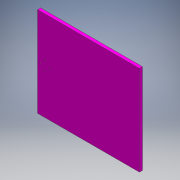
# Autodesk Inventor part: plaque
Saved by Autodesk Inventor 2017 (Build 210142000, 142)
## iProperties
Created: 2017-04-16
Part Number: plaque
Material: Generic
Document SubType Name: Modeling
Designer: franc
Density: 1 g/cm^3
Appearance: Default
Author: franc
Autodesk Inventor part; units mm, degrees
ref_plane "YZ Plane" through (0, 0, 0) normal (1, 0, 0) x (0, 1, 0)
ref_plane "XZ Plane" through (0, 0, 0) normal (0, 1, 0) x (-1, 0, 0)
ref_plane "XY Plane" through (0, 0, 0) normal (0, 0, 1) x (1, 0, 0)
sketch "Sketch1" plane through (0, 0, 0) normal (0, 1, 0) x (-1, 0, 0)
  line L0 (34, 64.6479) -> (-136, 64.6479)
  line L1 (-136, 64.6479) -> (-136, -85.3521)
  line L2 (-136, -85.3521) -> (34, -85.3521)
  line L3 (34, -85.3521) -> (34, 64.6479)
  circle A0 centre (29.5, -10.3521) radius 1
  circle A1 centre (13.5, -10.3521) radius 1
  circle A2 centre (21.5, -18.3521) radius 1
  circle A3 centre (21.5, -2.3521) radius 1
  point P0 (0, 0)
  dimension "d0" = 150
  dimension "d1" = 170
  dimension "d4" = 75
  dimension "d5" = 4.5
  dimension "d6" = 2
  dimension "d16" = 16
  dimension "d17" = 2
  dimension "d18" = 75
  dimension "d19" = 2
  dimension "d20" = 8
  dimension "d21" = 8
  dimension "d22" = 2
  dimension "d23" = 8
  dimension "d24" = 8
  constraints: 8 end point, 4 centre point, 2 parallel, 1 horizontal, 1 perpendicular
  measures "d0" distance of L2.end L0.start
  measures "d1" distance of L0.start L0.end
  measures "d4" distance from line of L0 A0.centre
  measures "d5" distance from line of A0.centre L3
  measures "d6" diameter of A0
  measures "d16" distance of A1.centre A0.centre
  measures "d17" diameter of A1
  measures "d18" distance from line of L0 A1.centre
  measures "d19" diameter of A2
  measures "d20" horizontal distance of A2.centre A0.centre
  measures "d21" horizontal distance of A2.centre A0.centre
  measures "d22" diameter of A3
  measures "d23" horizontal distance of A3.centre A0.centre
  measures "d24" horizontal distance of A0.centre A3.centre
extrude "Extrusion1" add sketch "Sketch1" along normal blind 5
body "Solid1"
